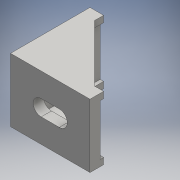
# Autodesk Inventor part: 3030 Corner Bracket External
Saved by Autodesk Inventor 2016 (Build 200138000, 138)
## iProperties
Created: 2017-04-11
Part Number: 3030 Corner Bracket External
Material: Generic
Document SubType Name: Modeling
Designer: Scott
Density: 1 g/cm^3
Appearance: Default
Author: Scott
## iProperties of the stored document 3030 Corner Bracket External_3DPrint.ipt
Created: 2017-04-15
Part Number: 3030 Corner Bracket External_3DPrint
Material: Generic
Document SubType Name: Modeling
Designer: Scott
Density: 1 g/cm^3
Appearance: Default
Author: Scott
Autodesk Inventor part; units mm, degrees
ref_plane "YZ Plane" through (0, 0, 0) normal (1, 0, 0) x (0, 1, 0)
ref_plane "XZ Plane" through (0, 0, 0) normal (0, 1, 0) x (-1, 0, 0)
ref_plane "XY Plane" through (0, 0, 0) normal (0, 0, 1) x (1, 0, 0)
sketch "Sketch1" plane through (0, 0, 0) normal (0, 0, 1) x (1, 0, 0)
  line L0 (0, 0) -> (35, 0)
  line L1 (35, 0) -> (35, 4.5)
  line L2 (35, 4.5) -> (4.5, 4.5)
  line L3 (4.5, 4.5) -> (4.5, 35)
  line L4 (4.5, 35) -> (0, 35)
  line L5 (0, 35) -> (0, 0)
  dimension "d0" = 35
  dimension "d1" = 35
  dimension "d2" = 4.5
  dimension "d3" = 4.5
  constraints: 12 end point, 4 perpendicular, 1 horizontal, 1 parallel
  measures "d0" distance of L0.start L0.end
  measures "d1" distance of L4.end L0.start
  measures "d2" distance of L3.end L4.end
  measures "d3" distance of L0.end L1.end
extrude "Extrusion1" add sketch "Sketch1" along normal mid plane 28
sketch "Sketch2" plane through (0, 0, 14) normal (0, 0, 1) x (1, 0, 0)
  line L0 (0, 0) -> (35, 0) projected
  line L1 (35, 0) -> (35, 4.5) projected
  line L2 (35, 4.5) -> (4.5, 4.5) projected
  line L3 (4.5, 4.5) -> (4.5, 35) projected
  line L4 (4.5, 35) -> (0, 35) projected
  line L5 (0, 35) -> (0, 0) projected
  line L6 (4.5, 35) -> (6, 35)
  line L7 (6, 35) -> (6, 31)
  line L8 (6, 31) -> (31, 6)
  line L9 (31, 6) -> (35, 6)
  line L10 (35, 4.5) -> (4.5, 4.5) projected
  line L11 (35, 6) -> (35, 4.5)
  dimension "d6" = 45
  dimension "d7" = 1.5
  dimension "d8" = 1.5
  dimension "d9" = 4
  constraints: 10 end point, 2 perpendicular, 1 horizontal, 1 parallel
  measures "d6" angle of L2 L8
  measures "d7" distance of L9.end L1.end
  measures "d8" distance of L3.end L6.end
  measures "d9" distance of L6.end L7.end
extrude "Extrusion2" add sketch "Sketch2" against normal blind 2.8 contours L2 L3 L6 L7 L8 L9 L11
mirror "Mirror1" about plane through (0, 0, 0) normal (0, 0, 1) of "Extrusion2"
sketch "Sketch3" plane through (0, 0, 14) normal (-1, 0, 0) x (0, 0, 1)
  line L0 (0, 0) -> (-28, 0) projected
  line L1 (0, 35) -> (0, 0) projected
  line L2 (-28, 35) -> (0, 35) projected
  line L3 (-28, 0) -> (-28, 35) projected
  line L4 (-25.2, 35) -> (-2.8, 35) construction
  line L5 (-14, 35) -> (-14, 0) construction
  line L6 (-14, 21.5) -> (-14, 13.5)
  line L7 (-17.5, 21.5) -> (-17.5, 13.5)
  line L8 (-10.5, 13.5) -> (-10.5, 21.5)
  arc A0 (-10.5, 21.5) -> (-17.5, 21.5) centre (-14, 21.5) ccw
  arc A1 (-17.5, 13.5) -> (-10.5, 13.5) centre (-14, 13.5) ccw
  point P0 (-14, 17.5)
  point P1 (-14, 17.5)
  dimension "d12" = 8
  dimension "d13" = 3.5
  constraints: 10 end point, 4 point on circle, 4 tangent, 3 midpoint, 2 centre point, 2 point on line, 1 coincident, 1 parallel, 1 vertical
  measures "d12" distance of L8.start L8.end
  measures "d13" radius of A0
extrude "Extrusion3" cut sketch "Sketch3" against normal through all contours A0 L8 A1 L7
sketch "Sketch4" plane through (0, 0, 14) normal (0, -1, 0) x (1, 0, 0)
  line L0 (35, -28) -> (35, 0) projected
  line L1 (0, 0) -> (35, 0) projected
  line L2 (0, 0) -> (0, -28) projected
  line L3 (35, -28) -> (0, -28) projected
  line L4 (0, -14) -> (35, -14) construction
  line L5 (13.5, -14) -> (21.5, -14) construction
  line L6 (13.5, -17.5) -> (21.5, -17.5)
  line L7 (21.5, -10.5) -> (13.5, -10.5)
  arc A0 (13.5, -10.5) -> (13.5, -17.5) centre (13.5, -14) ccw
  arc A1 (21.5, -17.5) -> (21.5, -10.5) centre (21.5, -14) ccw
  point P0 (17.5, -14)
  point P1 (17.5, -14)
  dimension "d16" = 8
  dimension "d17" = 3.5
  constraints: 10 end point, 4 point on circle, 4 tangent, 3 midpoint, 2 centre point, 2 point on line, 1 coincident, 1 parallel
  measures "d16" distance of L7.start L7.end
  measures "d17" radius of A1
extrude "Extrusion4" cut sketch "Sketch4" against normal through all contours A0 L7 A1 L6
body "Solid1"
